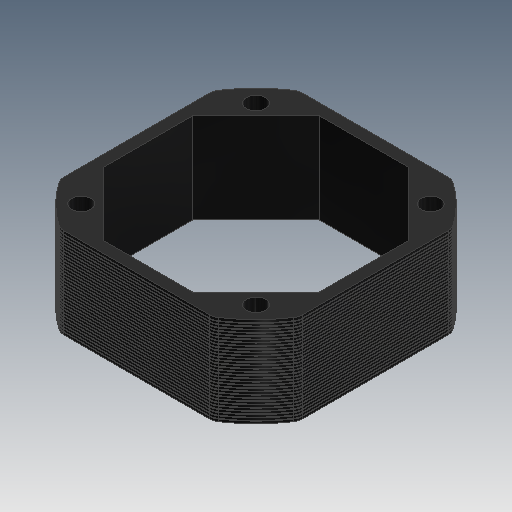
# Autodesk Inventor part: Nema 17 Central Spacer
Saved by Autodesk Inventor 2020.2 (Build 242310000, 310)
## iProperties
Created: 2020-01-17
Part Number: Nema 17 Central Spacer
Material: Iron, Ductile
Document SubType Name: Modeling
Designer: james
Density: 7.15 g/cm^3
Appearance: Smooth - Black
Mass: 49.8826 g
Surface Area: 69.5118 cm^2
Volume: 6.97658 cm^3
Author: james
Autodesk Inventor part; units mm, degrees
ref_plane "YZ Plane" through (0, 0, 0) normal (1, 0, 0) x (0, 1, 0)
ref_plane "XZ Plane" through (0, 0, 0) normal (0, 1, 0) x (-1, 0, 0)
sketch "Sketch11" plane through (0, 0, 0) normal (0, 1, 0) x (-1, 0, 0)
  line L0 (-13.5626, 21.15) -> (13.5626, 21.15)
  line L1 (21.15, 13.5626) -> (21.15, -13.5626)
  line L2 (13.5626, -21.15) -> (-13.5626, -21.15)
  line L3 (-21.15, -13.5626) -> (-21.15, 13.5626)
  line L4 (-21.15, 21.15) -> (21.15, -21.15) construction
  line L5 (21.15, 21.15) -> (-21.15, -21.15) construction
  line L6 (7.9322, -19.15) -> (-7.9322, -19.15)
  line L7 (-7.9322, -19.15) -> (-19.15, -7.9322)
  line L8 (-19.15, -7.9322) -> (-19.15, 7.9322)
  line L9 (-19.15, 7.9322) -> (-7.9322, 19.15)
  line L10 (-7.9322, 19.15) -> (7.9322, 19.15)
  line L11 (7.9322, 19.15) -> (19.15, 7.9322)
  line L12 (19.15, 7.9322) -> (19.15, -7.9322)
  line L13 (19.15, -7.9322) -> (7.9322, -19.15)
  arc A0 (13.5626, -21.15) -> (21.15, -13.5626) centre (0, 0) ccw
  arc A1 (21.15, 13.5626) -> (13.5626, 21.15) centre (0, 0) ccw
  arc A2 (-13.5626, 21.15) -> (-21.15, 13.5626) centre (0, 0) ccw
  arc A3 (-21.15, -13.5626) -> (-13.5626, -21.15) centre (0, 0) ccw
  point P0 (0, 0)
  dimension "d82" = 42.3
  dimension "d83" = 42.3
  dimension "d84" = 38.3
  dimension "d86" = 25.125
  constraints: 28 end point, 8 point on circle, 8 point on line, 4 centre point, 3 concentric, 2 coincident, 2 midpoint, 2 parallel, 1 horizontal, 1 perpendicular, 1 vertical, 17 other
  measures "d82" distance between parallel lines of L3 L1
  measures "d83" distance between parallel lines of L0 L2
  measures "d84" distance between parallel lines of L10 L6
  measures "d86" radius of A0
extrude "Extrusion7" add sketch "Sketch11" along normal mid plane 16
sketch "Sketch12" plane through (0, 8, 0) normal (0, 1, 0) x (1, 0, 0)
  line L0 (15.5, -15.5) -> (-15.5, -15.5) construction
  line L1 (-15.5, -15.5) -> (-15.5, 15.5) construction
  line L2 (-15.5, 15.5) -> (15.5, 15.5) construction
  line L3 (15.5, 15.5) -> (15.5, -15.5) construction
  line L4 (15.5, -15.5) -> (-15.5, 15.5) construction
  line L5 (-15.5, -15.5) -> (15.5, 15.5) construction
  point P0 (0, 0)
  point P1 (15.5, 15.5)
  point P2 (-15.5, -15.5)
  dimension "d89" = 31
  dimension "d90" = 31
  constraints: 12 end point, 4 coincident, 2 midpoint, 2 parallel, 1 horizontal, 1 perpendicular
  measures "d89" distance of L1.end L2.end
  measures "d90" distance of L0.end L1.end
hole "Hole5" at (-15.5, 8, -15.5) at (15.5, 8, -15.5) at (15.5, 8, 15.5) at (-15.5, 8, 15.5) direction (0, -1, 0) diameter 3.4 end through all clearance for "Flat Head Machine Screw" size "M3" standard "Ansi Metric M Profile"
fillet "Fillet8" radius 2 8 edges at (-21.15, 0, 13.5626) (-13.5626, 0, 21.15) (13.5626, 0, 21.15) (21.15, 0, 13.5626) (21.15, 0, -13.5626) (13.5626, 0, -21.15) (-13.5626, 0, -21.15) (-21.15, 0, -13.5626)
ref_plane "Work Plane6" through (0, 7.5, 0) normal (0, 1, 0) x (1, 0, 0)
sketch "Sketch13" plane through (0, 7.5, 0) normal (0, 1, 0) x (1, 0, 0)
  arc A0 (-20.8062, 14.0843) -> (-21.15, 12.9631) centre (-19.15, 12.9631) ccw projected
  line L0 (-21.15, 12.9631) -> (-21.15, -12.9631) projected
  arc A1 (-21.15, -12.9631) -> (-20.8062, -14.0843) centre (-19.15, -12.9631) ccw projected
  arc A2 (-20.8062, -14.0843) -> (-14.0843, -20.8062) centre (0, 0) ccw projected
  arc A3 (-14.0843, -20.8062) -> (-12.9631, -21.15) centre (-12.9631, -19.15) ccw projected
  line L1 (-12.9631, -21.15) -> (12.9631, -21.15) projected
  arc A4 (12.9631, -21.15) -> (14.0843, -20.8062) centre (12.9631, -19.15) ccw projected
  arc A5 (14.0843, -20.8062) -> (20.8062, -14.0843) centre (0, 0) ccw projected
  arc A6 (20.8062, -14.0843) -> (21.15, -12.9631) centre (19.15, -12.9631) ccw projected
  line L2 (21.15, -12.9631) -> (21.15, 12.9631) projected
  arc A7 (21.15, 12.9631) -> (20.8062, 14.0843) centre (19.15, 12.9631) ccw projected
  arc A8 (20.8062, 14.0843) -> (14.0843, 20.8062) centre (0, 0) ccw projected
  arc A9 (14.0843, 20.8062) -> (12.9631, 21.15) centre (12.9631, 19.15) ccw projected
  line L3 (12.9631, 21.15) -> (-12.9631, 21.15) projected
  arc A10 (-12.9631, 21.15) -> (-14.0843, 20.8062) centre (-12.9631, 19.15) ccw projected
  arc A11 (-14.0843, 20.8062) -> (-20.8062, 14.0843) centre (0, 0) ccw projected
  arc A12 (14.0282, -20.7234) -> (20.7234, -14.0282) centre (0, 0) ccw
  arc A13 (12.9631, -21.05) -> (14.0282, -20.7234) centre (12.9631, -19.15) ccw
  line L4 (12.9631, -21.05) -> (-12.9631, -21.05)
  arc A14 (-14.0282, -20.7234) -> (-12.9631, -21.05) centre (-12.9631, -19.15) ccw
  arc A15 (-20.7234, -14.0282) -> (-14.0282, -20.7234) centre (0, 0) ccw
  arc A16 (-21.05, -12.9631) -> (-20.7234, -14.0282) centre (-19.15, -12.9631) ccw
  line L5 (-21.05, -12.9631) -> (-21.05, 12.9631)
  arc A17 (-20.7234, 14.0282) -> (-21.05, 12.9631) centre (-19.15, 12.9631) ccw
  arc A18 (-14.0282, 20.7234) -> (-20.7234, 14.0282) centre (0, 0) ccw
  arc A19 (-12.9631, 21.05) -> (-14.0282, 20.7234) centre (-12.9631, 19.15) ccw
  line L6 (-12.9631, 21.05) -> (12.9631, 21.05)
  arc A20 (14.0282, 20.7234) -> (12.9631, 21.05) centre (12.9631, 19.15) ccw
  arc A21 (20.7234, 14.0282) -> (14.0282, 20.7234) centre (0, 0) ccw
  arc A22 (21.05, 12.9631) -> (20.7234, 14.0282) centre (19.15, 12.9631) ccw
  line L7 (21.05, 12.9631) -> (21.05, -12.9631)
  arc A23 (20.7234, -14.0282) -> (21.05, -12.9631) centre (19.15, -12.9631) ccw
  point P0 (0, 0)
  dimension "d100" = 0.1
  constraints: 24 point on circle, 12 centre point, 8 end point, 15 other
  measures "d100" radial gap between concentric circles of A5 A12
extrude "Extrusion8" cut sketch "Sketch13" against normal blind 0.1
pattern_linear "Rectangular Pattern1" count 31 spacing 0.5 along (0, -1, 0) of "Extrusion8"
body "Solid6"
